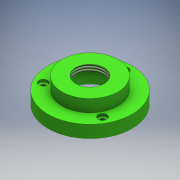
# Autodesk Inventor part: cylindricalObjectiveHolder
Saved by Autodesk Inventor 2016 (Build 200138000, 138)
## iProperties
Created: 2016-03-08
Part Number: cylindricalObjectiveHolder
Material: Generic
Document SubType Name: Modeling
Designer: sims01
Density: 1 g/cm^3
Appearance: Default
Author: sims01
Autodesk Inventor part; units mm, degrees
ref_plane "YZ Plane" through (0, 0, 0) normal (1, 0, 0) x (0, 1, 0)
ref_plane "XZ Plane" through (0, 0, 0) normal (0, 1, 0) x (-1, 0, 0)
ref_plane "XY Plane" through (0, 0, 0) normal (0, 0, 1) x (1, 0, 0)
sketch "Sketch3" plane through (0, 0, 0) normal (0, 0, 1) x (1, 0, 0)
  circle A0 centre (0, 0) radius 33.75
  dimension "d7" = 67.5
  constraints: 1 centre point, 1 coincident
  measures "d7" diameter of A0
extrude "baseExtrusion" add sketch "Sketch3" along normal blind 10
sketch "Sketch4" plane through (0, 0, 10) normal (0, 0, 1) x (1, 0, 0)
  circle A0 centre (0, 0) radius 22.5
  dimension "d10" = 45
  constraints: 1 centre point, 1 coincident
  measures "d10" diameter of A0
extrude "objectiveMountExtrusion" add sketch "Sketch4" along normal blind 10
sketch "Sketch5" plane through (0, 0, 20) normal (0, 0, 1) x (1, 0, 0)
  point P0 (0, 0)
  point P1 (0, 0)
  constraints: 1 coincident
hole "objectiveThread" at (0, 0, 20) direction (0, 0, -1) diameter 22.835 end through all thread size "M25x2" class "6H" standard "ISO Metric profile"
sketch "Sketch6" plane through (0, 0, 0) normal (0, 0, -1) x (-1, 0, 0)
  circle A0 centre (0, 0) radius 20
  dimension "d20" = 40
  constraints: 1 centre point, 1 coincident
  measures "d20" diameter of A0
extrude "objectiveClearance" cut sketch "Sketch6" against normal blind 14.7
sketch "Sketch7" plane through (0, 0, 10) normal (0, 0, 1) x (1, 0, 0)
  point P0 (0, 0)
  point P1 (0, 27.5)
  point P2 (-23.8157, -13.75)
  point P3 (23.8157, -13.75)
  dimension "d23" = 27.5
  dimension "d26" = 360
  constraints: 4 other
  measures "d23" distance of point (0, 0) point (0, 27.5)
hole "holeMounts" at (0, 27.5, 10) at (-23.8157, -13.75, 10) at (23.8157, -13.75, 10) direction (0, 0, -1) diameter 3.242 end through all counterbore diameter 7 counterbore depth 2 thread size "M4x0.7" class "6H" standard "ISO Metric profile"
body "Solid2"
